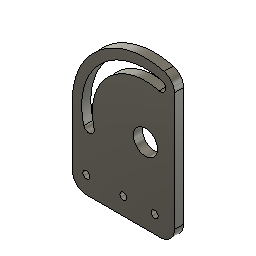
hinge-plate v1 (Autodesk Fusion 360 design; units mm, degrees)
Autodesk Fusion 360 part; units mm, degrees
sketch "Sketch1" plane through (0, 0, 0) normal (0, 0, 1) x (1, 0, 0)
  circle A0 centre (0, 0) radius 10.5
  circle A1 centre (0, 0) radius 4
  arc A2 (11.8123, 44.4575) -> (-44.4575, -11.8123) centre (0, 0) ccw
  arc A3 (14.1876, 53.3973) -> (-53.3973, -14.1876) centre (0, 0) ccw
  arc A4 (-53.3973, -14.1876) -> (-44.4575, -11.8123) centre (-48.9274, -13) ccw
  arc A5 (11.8123, 44.4575) -> (14.1876, 53.3973) centre (13, 48.9274) ccw
  line L0 (25, 58.0996) -> (25, -65)
  line L1 (-63.25, -65) -> (25, -65)
  line L2 (-63.25, 0) -> (-63.25, -65)
  arc A6 (25, 58.0996) -> (-63.25, 0) centre (0, 0) ccw
  circle A7 centre (-51.25, -50) radius 3
  circle A8 centre (-19.125, -50) radius 3
  circle A9 centre (8, -50) radius 3
  dimension "d1" = 21
  dimension "d2" = 8
  dimension "d3" = 92
  dimension "d4" = 110.5
  dimension "d5" = 9.25
  dimension "d6" = 9.25
  dimension "d9" = 126.5
  dimension "d10" = 25
  dimension "d11" = 12
  dimension "d13" = 6
  dimension "d14" = 6
  dimension "d15" = 6
  dimension "d16" = 15
  dimension "d18" = 15
  dimension "d19" = 15
  dimension "d21" = 12
  dimension "d22" = 17
  dimension "d29" = 65
  dimension "d30" = 50.625
  dimension "d33" = 44.125
  dimension "d34" = 13
  constraint coincident A0.centre A1.centre
  constraint concentric A0 A1
  constraint concentric A0 A2
  constraint concentric A0 A3
  constraint concentric A2 A6
  constraint vertical L0
  constraint parallel L0 L2
  constraint tangent L2 A6
  constraint perpendicular L1 L2
  measures "d1" diameter of A0
  measures "d2" diameter of A1
  measures "d3" diameter of A2
  measures "d4" diameter of A3
  measures "d5" diameter of A5
  measures "d6" diameter of A4
  measures "d9" diameter of A6
  measures "d10" distance of A0.centre L0
  measures "d11" distance of A5.centre L0
  measures "d13" diameter of A7
  measures "d14" diameter of A8
  measures "d15" diameter of A9
  measures "d16" distance of L1 A9.centre
  measures "d18" distance of L1 A8.centre
  measures "d19" distance of L1 A7.centre
  measures "d21" distance of L2 A7.centre
  measures "d22" distance of L0 A9.centre
  measures "d29" distance of A0.centre L1
  measures "d30" distance of A0.centre A5.centre
  measures "d33" distance of L0 A8.centre
  measures "d34" vertical distance of A4.centre A0.centre
extrude "Extrude1" add sketch "Sketch1" along normal blind 8 contours L0 L1 L2 A6
fillet "Fillet1" radius 12 3 edges at (-63.25, -65, 4) (25, -65, 4) (25, 58.0996, 4)
equation "d4 = d3 + 18.5 mm"
equation "d5 = d6"
equation "d6 = ( d4 - d3 ) / 2"
equation "d9 = d4 + 16 mm"
equation "d18 = d16"
equation "d19 = d16"
equation "d21 = d11"
equation "d22 = d11 + 5 mm"
equation "d33 = ( ( d9 / 2 ) + d10 ) / 2"
equation "d34 = d10 - d11"
